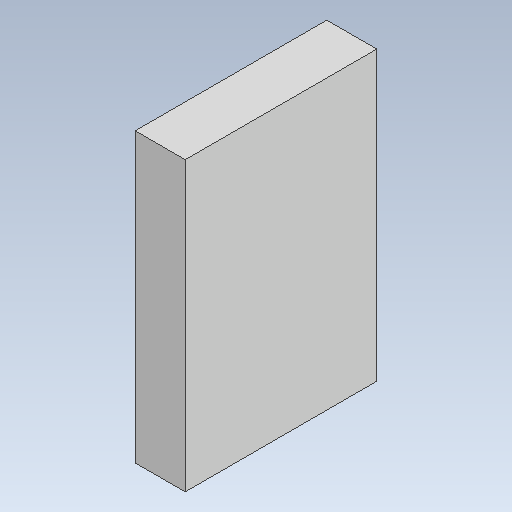
# Autodesk Inventor part: Body
Saved by Autodesk Inventor 2020 (Build 240168000, 168)
## iProperties
Created: 2020-06-06
Part Number: Body
Material: Generic
Document SubType Name: Modeling
Designer: user
Density: 1 g/cm^3
Appearance: Default
Author: user
Autodesk Inventor part; units mm, degrees
ref_plane "YZ Plane" through (0, 0, 0) normal (1, 0, 0) x (0, 1, 0)
ref_plane "XZ Plane" through (0, 0, 0) normal (0, 1, 0) x (-1, 0, 0)
ref_plane "XY Plane" through (0, 0, 0) normal (0, 0, 1) x (1, 0, 0)
sketch "Sketch1" plane through (0, 0, 0) normal (0, 1, 0) x (-1, 0, 0)
  line L0 (10.8401, 18.8589) -> (2.1401, 18.8589)
  line L1 (2.1401, 18.8589) -> (2.1401, -14.4411)
  line L2 (2.1401, -14.4411) -> (10.8401, -14.4411)
  line L3 (10.8401, -14.4411) -> (10.8401, 18.8589)
  point P0 (0, 0)
  dimension "d0" = 33.3
  dimension "d1" = 8.7
  constraints: 8 end point, 2 parallel, 1 horizontal, 1 perpendicular
  measures "d0" distance of L2.end L0.start
  measures "d1" distance of L1.end L2.end
extrude "Extrusion1" add sketch "Sketch1" along normal blind 50
sketch "Sketch2" plane through (0, 0, 0) normal (0, -1, 0) x (1, 0, 0)
  line L0 (-9.3401, 15.9589) -> (-4.6401, 15.9589)
  line L1 (-4.6401, 15.9589) -> (-4.6401, -11.5411)
  line L2 (-4.6401, -11.5411) -> (-9.3401, -11.5411)
  line L3 (-9.3401, -11.5411) -> (-9.3401, 15.9589)
  line L4 (-2.1401, 18.8589) -> (-2.1401, -14.4411) projected
  line L5 (-10.8401, 18.8589) -> (-2.1401, 18.8589) projected
  line L6 (-10.8401, -14.4411) -> (-10.8401, 18.8589) projected
  line L7 (-2.1401, -14.4411) -> (-10.8401, -14.4411) projected
  point P0 (0, 0)
  dimension "d4" = 2.5
  dimension "d5" = 2.9
  dimension "d6" = 1.5
  dimension "d7" = 2.9
  constraints: 8 end point, 2 parallel, 1 horizontal, 1 perpendicular
  measures "d4" distance between parallel lines of L4 L1
  measures "d5" distance between parallel lines of L5 L0
  measures "d6" distance between parallel lines of L6 L3
  measures "d7" distance between parallel lines of L7 L2
extrude "Extrusion2" cut sketch "Sketch2" against normal blind 10 contours L0 L1 L2 L3
equation "\"d4\" = ClipHeight"
equation "\"d5\" = ClipWidth"
equation "\"d7\" = d5"
equation "\"ClipHeight\" = 2.5"
equation "\"ClipWidth\" = 2.9"
body "Solid1"
